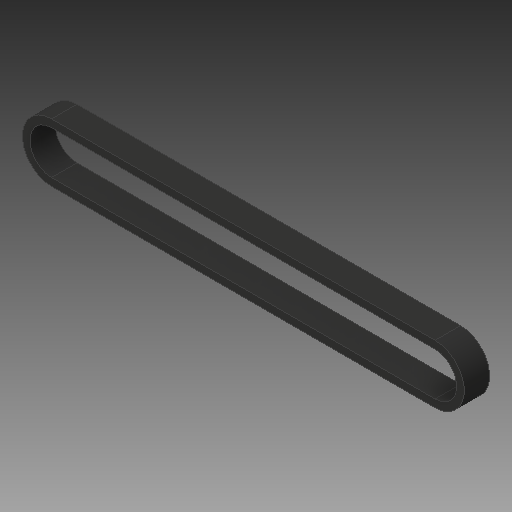
# Autodesk Inventor part: faja
Saved by Autodesk Inventor 2019 (Build 230136000, 136)
## iProperties
Created: 2020-02-22
Part Number: faja
Material: Rubber, Silicone
Document SubType Name: Modeling
Designer: Elías Sánchez
Density: 1.25 g/cm^3
Appearance: Rubber - Black
Description: -
Author: Elías Sánchez
Autodesk Inventor part; units mm, degrees
ref_plane "YZ Plane" through (0, 0, 0) normal (1, 0, 0) x (0, 1, 0)
ref_plane "XZ Plane" through (0, 0, 0) normal (0, 1, 0) x (-1, 0, 0)
ref_plane "XY Plane" through (0, 0, 0) normal (0, 0, 1) x (1, 0, 0)
sketch "Sketch1" plane through (0, 0, 0) normal (0, 0, 1) x (1, 0, 0)
  line L0 (-75.5, 11.5) -> (75.5, 11.5)
  line L1 (75.5, -11.5) -> (-75.5, -11.5)
  arc A0 (-75.5, 11.5) -> (-75.5, -11.5) centre (-75.5, 0) ccw
  arc A1 (75.5, -11.5) -> (75.5, 11.5) centre (75.5, 0) ccw
  line L2 (-75.5, 8.5) -> (75.5, 8.5)
  line L3 (-75.5, -8.5) -> (75.5, -8.5)
  arc A2 (-75.5, 8.5) -> (-75.5, -8.5) centre (-75.5, 0) ccw
  arc A3 (75.5, -8.5) -> (75.5, 8.5) centre (75.5, 0) ccw
  point P0 (0, 0)
  point P1 (0, 8.5)
  point P2 (0, 11.5)
  dimension "d0" = 151
  dimension "d1" = 23
  dimension "d2" = 3
  dimension "d3" = 3
  dimension "d4" = 11.5
  dimension "d5" = 8.5
  dimension "d7" = 8.5
  dimension "d8" = 151
  dimension "d9" = 151
  constraints: 8 end point, 8 point on circle, 4 centre point, 4 tangent, 3 horizontal, 2 midpoint, 2 vertical alignment, 1 horizontal alignment, 1 parallel
  measures "d0" distance of L1.start L1.end
  measures "d1" distance between parallel lines of L1 L0
  measures "d2" distance between parallel lines of L1 L3
  measures "d3" distance between parallel lines of L0 L2
  measures "d4" radius of A1
  measures "d5" radius of A3
  measures "d7" radius of A2
  measures "d8" distance of A1.centre A0.centre
  measures "d9" distance of A2.centre A3.centre
extrude "Extrusion1" add sketch "Sketch1" along normal blind 10
body "Solid1"
